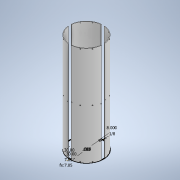
# Autodesk Inventor part: can
Saved by Autodesk Inventor 2021 (Build 250183000, 183)
## iProperties
Created: 2020-09-04
Part Number: can
Material: Generic
Document SubType Name: Modeling
Designer: dsouthall
Density: 1 g/cm^3
Appearance: Default
Author: dsouthall
Autodesk Inventor part; units mm, degrees
sketch "Sketch1" plane through (0, 0, 0) normal (0, 1, 0) x (-1, 0, 0)
  circle A0 centre (0, 0) radius 101.6
  circle A1 centre (0, 0) radius 98.425
  line L0 (0, 98.425) -> (0, -98.425) construction
  line L1 (0, 0) -> (12.080237, 97.68085) construction
  line L2 (0, 0) -> (-12.080237, 97.68085) construction
  line L3 (0, 0) -> (50.8, 87.988181) construction
  line L4 (0, 0) -> (87.988181, 50.8) construction
  dimension "OD" = 203.2
  dimension "thickness" = 3.175
  dimension "d13" = 7.05
  dimension "d15" = 7.05
  dimension "d88" = 30
  dimension "d89" = 30
  dimension "d90" = 0
  dimension "d91" = 0
  dimension "d119" = 0
  constraints: 10 end point, 6 point on circle, 2 centre point, 1 coincident, 1 vertical
  measures "OD" diameter of A0
  measures "thickness" radial gap between concentric circles of A1 A0
  measures "d13" angle of L1 L0
  measures "d15" angle of L0 L2
  measures "d88" angle of L3 L0
  measures "d89" angle of L4 L3
  measures "d90" distance of A0.centre point (0, 0)
  measures "d91" distance of point (0, 0) A0.centre
  measures "d119" distance from line of point (0, 0) L0
extrude "Extrusion1" add sketch "Sketch1" along normal blind 600
ref_plane "Work Plane1" through (0, 0, 101.6) normal (0, 0, 1) x (1, 0, 0)
sketch "Sketch2" plane through (0, 0, 101.6) normal (0, 0, 1) x (1, 0, 0)
  line L0 (-10, 600) -> (10, 600)
  line L1 (10, 600) -> (10, 0)
  line L2 (10, 0) -> (-10, 0)
  line L3 (-10, 0) -> (-10, 600)
  line L4 (101.6, 600) -> (-101.6, 600) projected
  line L5 (101.6, 0) -> (-101.6, 0) projected
  point P0 (0, 0)
  point P1 (0, 0)
  dimension "edge_height" = 0
  dimension "d5" = 0
  dimension "slot_width" = 20
  dimension "d7" = 10
  constraints: 8 end point, 2 parallel, 1 horizontal, 1 midpoint, 1 perpendicular
  measures "edge_height" distance between parallel lines of L4 L0
  measures "d5" distance between parallel lines of L5 L2
  measures "slot_width" distance between parallel lines of L1 L3
  measures "d7" distance from line of point (0, 0) L1
extrude "Extrusion2" cut sketch "Sketch2" against normal blind 12.7
pattern_circular "Circular Pattern1" count 4 over 360 about axis through (0, 0, 0) along (0, 1, 0) of "Extrusion2"
ref_plane "Central Plane" through (0, 300, 0) normal (0, -1, 0) x (1, 0, 0)
ref_plane "Offset Plane A" through (0, 296.002659, 0) normal (0, -1, 0) x (1, 0, 0)
ref_plane "Offset Plane B" through (0, 303.997341, 0) normal (0, -1, 0) x (1, 0, 0)
ref_plane "Work Plane5" through (-12.469922, 296.002659, 100.831845) normal (-0.1227355, 0, 0.9924394) x (0, -1, 0)
ref_plane "Work Plane6" through (12.469922, 303.997341, 100.831845) normal (0.1227355, 0, 0.9924394) x (0, 1, 0)
hole "Hole1" at (12.469922, 303.997341, 100.831845) direction (-0.1227355, 0, -0.9924394) diameter 2.4384 depth 25.4 countersink diameter 4.699 countersink angle 82 clearance for "Flat Head Machine Screw (82)" size "#2" standard "Ansi Unified Screw Threads"
hole "Hole2" at (-12.469922, 296.002659, 100.831845) direction (0.1227355, 0, -0.9924394) diameter 2.4384 depth 25.4 tip angle 118 countersink diameter 4.699 countersink angle 82 clearance for "Flat Head Machine Screw (82)" size "#2" standard "Ansi Unified Screw Threads"
pattern_circular "Circular Pattern3" count 4 over 360 about axis through (0, 600, 0) along (0, -1, 0) of "Hole1", "Hole2"
ref_plane "plane for insert hole 1" through (-50.8, 0, 87.988181) normal (-0.5, 0, 0.8660254) x (0, -1, 0)
sketch "Sketch7" plane through (-50.8, 0, 87.988181) normal (-0.5, 0, 0.8660254) x (0, -1, 0)
  line L0 (-600, 41.893084) -> (-600, -82.56095)
  point P0 (0, 0)
  point P1 (-300, 0)
  point P2 (-595, 0)
  point P3 (-5, 0)
  dimension "d92" = 0
  dimension "d93" = 300
  dimension "d124" = 0
  dimension "d125" = 0
  dimension "d126" = 5
  dimension "d127" = 5
  measures "d92" vertical distance of point (0, 0) point (-300, 0)
  measures "d93" distance of point (0, 0) point (-300, 0)
  measures "d124" vertical distance of point (0, 0) point (-5, 0)
  measures "d125" vertical distance of point (0, 0) point (-595, 0)
  measures "d126" distance of point (0, 0) point (-5, 0)
  measures "d127" distance from line of L0 point (-595, 0)
ref_plane "plane for insert hole 2" through (-87.988181, 0, 50.8) normal (-0.8660254, 0, 0.5) x (0, -1, 0)
sketch "Sketch8" plane through (-87.988181, 0, 50.8) normal (-0.8660254, 0, 0.5) x (0, -1, 0)
  line L0 (-600, 82.56095) -> (-600, -41.893084) construction
  point P0 (0, 0)
  point P1 (-300, 0)
  point P2 (-595, 0)
  point P3 (-5, 0)
  dimension "d94" = 0
  dimension "d95" = 300
  dimension "d120" = 0
  dimension "d121" = 0
  dimension "d122" = 5
  dimension "d123" = 5
  measures "d94" vertical distance of point (0, 0) point (-300, 0)
  measures "d95" distance of point (0, 0) point (-300, 0)
  measures "d120" vertical distance of point (0, 0) point (-5, 0)
  measures "d121" vertical distance of point (0, 0) point (-595, 0)
  measures "d122" distance of point (0, 0) point (-5, 0)
  measures "d123" distance from line of L0 point (-595, 0)
hole "insert hole 2" at (-87.988181, 300, 50.8) direction (0.8660254, 0, -0.5) diameter 3.2766 depth 8.8646 tip angle 118 countersink diameter 5.715 countersink angle 82 clearance for "Flat Head Machine Screw (82)" size "#4" standard "Ansi Unified Screw Threads"
hole "insert hole 1" at (-50.8, 300, 87.988181) direction (0.5, 0, -0.8660254) diameter 3.2766 depth 8.8646 tip angle 118 countersink diameter 5.715 countersink angle 82 clearance for "Flat Head Machine Screw (82)" size "#4" standard "Ansi Unified Screw Threads"
pattern_circular "Circular Pattern7" count 4 over 360 about axis through (0, 0, 0) along (0, 1, 0) of "insert hole 2"
pattern_circular "Circular Pattern9" count 4 over 360 about axis through (0, 0, 0) along (0, 1, 0) of "insert hole 1"
hole "Hole8" at (-87.988181, 5, 50.8) at (-87.988181, 595, 50.8) direction (0.8660254, 0, -0.5) diameter 3.2766 depth 8.8646 tip angle 118 countersink diameter 5.715 countersink angle 82 clearance for "Flat Head Machine Screw (82)" size "#4" standard "Ansi Unified Screw Threads"
hole "Hole9" at (-50.8, 5, 87.988181) at (-50.8, 595, 87.988181) direction (0.5, 0, -0.8660254) diameter 3.2766 depth 8.8646 tip angle 118 countersink diameter 5.715 countersink angle 82 clearance for "Flat Head Machine Screw (82)" size "#4" standard "Ansi Unified Screw Threads"
pattern_circular "Circular Pattern10" count 4 over 360 about axis through (0, 600, 0) along (0, -1, 0) of "Hole8"
pattern_circular "Circular Pattern11" count 4 over 360 about axis through (0, 600, 0) along (0, -1, 0) of "Hole9"
equation "\"d15\" = d13"
equation "\"d7\" = 0.5 * slot_width"
equation "\"d93\" = 0.5 * height"
equation "\"d126\" = d122"
equation "\"d127\" = d122"
equation "\"d95\" = 0.5 * height"
equation "\"d123\" = d122"
equation "\"height\" = 600"
body "Solid1"
